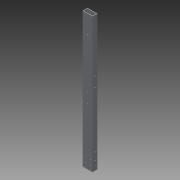
# Autodesk Inventor part: SuperSuperStructure
Saved by Autodesk Inventor 2013 (Build 170138000, 138)
## iProperties
Created: 2014-01-18
Part Number: SuperSuperStructure
Material: Generic
Document SubType Name: Modeling
Designer: 215152
Density: 1 g/cm^3
Author: 215152
Autodesk Inventor part; units mm, degrees
ref_plane "YZ Plane" through (0, 0, 0) normal (1, 0, 0) x (0, 1, 0)
ref_plane "XZ Plane" through (0, 0, 0) normal (0, 1, 0) x (-1, 0, 0)
ref_plane "XY Plane" through (0, 0, 0) normal (0, 0, 1) x (1, 0, 0)
sketch "Sketch1" plane through (0, 0, 0) normal (0, 1, 0) x (-1, 0, 0)
  line L0 (-25.4, -12.7) -> (25.4, -12.7)
  line L1 (25.4, -12.7) -> (25.4, 12.7)
  line L2 (25.4, 12.7) -> (-25.4, 12.7)
  line L3 (-25.4, 12.7) -> (-25.4, -12.7)
  line L4 (-25.4, -12.7) -> (25.4, 12.7) construction
  line L5 (25.4, -12.7) -> (-25.4, 12.7) construction
  line L6 (22.225, -9.525) -> (-22.225, -9.525)
  line L7 (-22.225, -9.525) -> (-22.225, 9.525)
  line L8 (-22.225, 9.525) -> (22.225, 9.525)
  line L9 (22.225, 9.525) -> (22.225, -9.525)
  line L10 (22.225, -9.525) -> (-22.225, 9.525) construction
  line L11 (-22.225, -9.525) -> (22.225, 9.525) construction
  point P0 (0, 0)
  dimension "d0" = 50.8
  dimension "d1" = 25.4
  dimension "d2" = 44.45
  dimension "d3" = 19.05
  constraints: 24 end point, 4 midpoint, 4 parallel, 2 horizontal, 2 perpendicular
  measures "d0" distance of L2.end L1.end
  measures "d1" distance of L1.end L0.end
  measures "d2" distance of L7.end L8.end
  measures "d3" distance of L6.end L7.end
extrude "Extrusion1" add sketch "Sketch1" along normal blind 609.6
sketch "Sketch2" plane through (-25.4, 0, 12.7) normal (0, 0, 1) x (1, 0, 0)
  line L0 (0, 609.6) -> (25.4, 609.6)
  line L1 (25.4, 609.6) -> (25.4, 584.2)
  line L2 (25.4, 584.2) -> (0, 584.2)
  line L3 (0, 584.2) -> (0, 609.6)
  circle A0 centre (25.4, 584.2) radius 6.35
  point P0 (25.4, 0)
  dimension "d6" = 25.4
  dimension "d7" = 25.4
  dimension "d8" = 12.7
  constraints: 8 end point, 2 parallel, 1 centre point, 1 coincident, 1 horizontal, 1 perpendicular
  measures "d6" distance of L1.end L2.end
  measures "d7" distance of L0.end L1.end
  measures "d8" diameter of A0
extrude "Extrusion2" cut sketch "Sketch2" against normal blind 609.6 contours A0 L2 L1 | L1 L2 A0
sketch "Sketch3" plane through (-25.4, 0, 12.7) normal (0, 0, 1) x (1, 0, 0)
  line L0 (0, 0) -> (50.8, 0)
  line L1 (50.8, 0) -> (50.8, 50.8)
  line L2 (50.8, 50.8) -> (0, 50.8)
  line L3 (0, 50.8) -> (0, 0)
  line L4 (50.8, 50.8) -> (25.4, 50.8)
  line L5 (25.4, 50.8) -> (25.4, 0)
  line L6 (25.4, 0) -> (50.8, 0)
  line L7 (50.8, 0) -> (50.8, 50.8)
  line L8 (50.8, 0) -> (0, 0)
  line L9 (0, 0) -> (0, 25.4)
  line L10 (0, 25.4) -> (50.8, 25.4)
  line L11 (50.8, 25.4) -> (50.8, 0)
  line L12 (25.4, 25.4) -> (12.7, 25.4)
  line L13 (12.7, 25.4) -> (12.7, 38.1)
  line L14 (12.7, 38.1) -> (25.4, 38.1)
  line L15 (25.4, 38.1) -> (25.4, 25.4)
  line L16 (12.7, 38.1) -> (38.1, 38.1)
  line L17 (38.1, 38.1) -> (38.1, 12.7)
  line L18 (38.1, 12.7) -> (12.7, 12.7)
  line L19 (12.7, 12.7) -> (12.7, 38.1)
  circle A0 centre (12.7, 38.1) radius 3.175
  circle A1 centre (38.1, 38.1) radius 3.175
  circle A2 centre (38.1, 12.7) radius 3.175
  circle A3 centre (12.7, 12.7) radius 3.175
  dimension "d11" = 50.8
  dimension "d12" = 50.8
  dimension "d13" = 50.8
  dimension "d14" = 25.4
  dimension "d15" = 12.7
  dimension "d16" = 12.7
  dimension "d17" = 25.4
  dimension "d18" = 25.4
  dimension "d19" = 6.35
  dimension "d20" = 6.35
  dimension "d21" = 6.35
  dimension "d22" = 6.35
  constraints: 40 end point, 10 parallel, 5 horizontal, 5 perpendicular, 4 centre point, 4 coincident, 1 midpoint
  measures "d11" distance of L2.end L1.end
  measures "d12" distance of L1.end L0.end
  measures "d13" distance of L9.end L10.end
  measures "d14" distance of L8.end L9.end
  measures "d15" distance of L13.end L14.end
  measures "d16" distance of L12.end L13.end
  measures "d17" distance of L17.end L18.end
  measures "d18" distance of L16.end L17.end
  measures "d19" diameter of A0
  measures "d20" diameter of A1
  measures "d21" diameter of A2
  measures "d22" diameter of A3
extrude "Extrusion3" cut sketch "Sketch3" against normal blind 609.6 contours A2 L17 L18 | L18 L17 A2 | A3 L19 L18 | L18 L19 A3 | A0 L14 L13 | L13 L14 A0 | A1 L16 L17 | L17 L16 A1
sketch "Sketch4" plane through (0, 0, 0) normal (0, -1, 0) x (1, 0, 0)
  line L0 (22.225, 9.525) -> (22.225, -9.525) projected
  line L1 (22.225, -9.525) -> (-22.225, -9.525) projected
  line L2 (-22.225, -9.525) -> (-22.225, 9.525) projected
  line L3 (-22.225, 9.525) -> (22.225, 9.525) projected
  line L4 (25.4, -12.7) -> (-25.4, -12.7) projected
  line L5 (25.4, 12.7) -> (25.4, -12.7) projected
  line L6 (-25.4, 12.7) -> (25.4, 12.7) projected
  line L7 (-25.4, -12.7) -> (-25.4, 12.7) projected
  point P0 (0, 0)
extrude "Extrusion4" add sketch "Sketch4" along normal blind 12.7
sketch "Sketch5" plane through (25.4, 609.6, -12.7) normal (0, 0, -1) x (-1, 0, 0)
  circle A0 centre (12.7, -596.9) radius 3.175 projected
  line L0 (50.8, -622.3) -> (0, -622.3) projected
  line L1 (12.7, -596.9) -> (12.7, -615.95)
  line L2 (12.7, -596.9) -> (31.75, -596.9) construction
  line L3 (12.7, -615.95) -> (38.1, -615.95)
  circle A1 centre (12.7, -615.95) radius 2.54
  circle A2 centre (38.1, -615.95) radius 2.54
  point P0 (25.4, -609.6)
  dimension "d27" = 19.05
  dimension "d28" = 90
  dimension "d29" = 25.4
  dimension "d30" = 90
  dimension "d31" = 5.08
  dimension "d32" = 5.08
  constraints: 6 end point, 3 perpendicular, 2 centre point, 2 coincident, 1 horizontal
  measures "d27" distance of L1.start L1.end
  measures "d28" angle of L1 L2
  measures "d29" distance of L1.end L3.end
  measures "d30" angle of L3 L1
  measures "d31" diameter of A1
  measures "d32" diameter of A2
extrude "Extrusion5" cut sketch "Sketch5" against normal blind 25.4 contours A1 L3 L1 | L1 L3 A1 | A2
sketch "Sketch6" plane through (0, 609.6, 0) normal (0, 1, 0) x (1, 0, 0)
  line L0 (22.225, 9.525) -> (22.225, -9.525) projected
  line L1 (22.225, -9.525) -> (-22.225, -9.525) projected
  line L2 (-22.225, -9.525) -> (-22.225, 9.525) projected
  line L3 (-22.225, 9.525) -> (22.225, 9.525) projected
  line L4 (25.4, 12.7) -> (-25.4, 12.7) projected
  line L5 (-25.4, 12.7) -> (-25.4, -12.7) projected
  line L6 (-25.4, -12.7) -> (25.4, -12.7) projected
  line L7 (25.4, -12.7) -> (25.4, 12.7) projected
  point P0 (0, 0)
extrude "Extrusion6" add sketch "Sketch6" along normal blind 63.5
sketch "Sketch7" plane through (25.4, -12.7, 12.7) normal (1, 0, 0) x (0, 0, -1)
  line L0 (25.4, 685.8) -> (25.4, 0) projected
  line L1 (0, 685.8) -> (25.4, 685.8) projected
  line L2 (12.7, 685.8) -> (12.7, 419.1)
  line L3 (12.7, 685.8) -> (279.4, 685.8) construction
  circle A0 centre (12.7, 419.1) radius 3.175
  line L4 (12.7, 419.1) -> (12.7, 368.3)
  line L5 (12.7, 368.3) -> (12.7, 317.5)
  line L6 (12.7, 368.3) -> (63.5, 368.3) construction
  circle A1 centre (12.7, 368.3) radius 3.175
  circle A2 centre (12.7, 317.5) radius 3.175
  point P0 (12.7, 12.7)
  dimension "d37" = 266.7
  dimension "d38" = 90
  dimension "d39" = 6.35
  dimension "d40" = 50.8
  dimension "d41" = 50.8
  dimension "d42" = 90
  dimension "d43" = 6.35
  dimension "d44" = 6.35
  constraints: 10 end point, 3 centre point, 3 coincident, 3 perpendicular, 2 horizontal, 1 collinear, 1 midpoint, 1 parallel
  measures "d37" distance of L2.start L2.end
  measures "d38" angle of L2 L3
  measures "d39" diameter of A0
  measures "d40" distance of L4.start L4.end
  measures "d41" distance of L4.end L5.end
  measures "d42" angle of L5 L6
  measures "d43" diameter of A1
  measures "d44" diameter of A2
extrude "Extrusion8" cut sketch "Sketch7" against normal blind 50.8 contours A0 L4 L2 | L2 L4 A0 | A1 L5 L4 | L4 L5 A1
sketch "Sketch8" plane through (-25.4, -12.7, 12.7) normal (0, 0, 1) x (1, 0, 0)
  line L0 (50.8, 0) -> (50.8, 685.8) projected
  line L1 (0, 685.8) -> (50.8, 685.8) projected
  line L2 (25.4, 685.8) -> (25.4, 341.8078)
  line L3 (25.4, 685.8) -> (369.3922, 685.8) construction
  line L4 (25.4, 341.8078) -> (25.4, 291.0078)
  circle A0 centre (25.4, 291.0078) radius 3.175
  circle A1 centre (25.4, 341.8078) radius 3.175
  point P0 (25.4, 12.7)
  dimension "d49" = 343.9922
  dimension "d50" = 90
  dimension "d51" = 50.8
  dimension "d52" = 180
  dimension "d53" = 6.35
  dimension "d54" = 6.35
  constraints: 6 end point, 2 centre point, 2 coincident, 2 parallel, 1 horizontal, 1 midpoint, 1 perpendicular
  measures "d49" distance of L2.start L2.end
  measures "d50" angle of L2 L3
  measures "d51" distance of L2.end L4.end
  measures "d52" angle of L4 L2
  measures "d53" diameter of A0
  measures "d54" diameter of A1
extrude "Extrusion9" cut sketch "Sketch8" against normal blind 50.8
sketch "Sketch9" plane through (25.4, -12.7, 12.7) normal (1, 0, 0) x (0, 0, -1)
  line L0 (25.4, 0) -> (0, 0) projected
  line L1 (12.7, 0) -> (12.7, 84.1502)
  line L2 (12.7, 84.1502) -> (12.7, 46.0502)
  line L3 (12.7, 84.1502) -> (50.8, 84.1502) construction
  point P0 (12.7, 12.7)
  dimension "d57" = 84.1502
  dimension "d58" = 38.1
  dimension "d59" = 90
  constraints: 6 end point, 2 coincident, 2 perpendicular, 1 collinear, 1 horizontal, 1 midpoint
  measures "d57" distance of L1.start L1.end
  measures "d58" distance of L1.end L2.end
  measures "d59" angle of L2 L3
hole "Hole1" at (25.4, 71.4502, 0) at (25.4, 33.3502, 0) direction (-1, 0, 0) diameter 6.35 end through all
body "Solid1"
